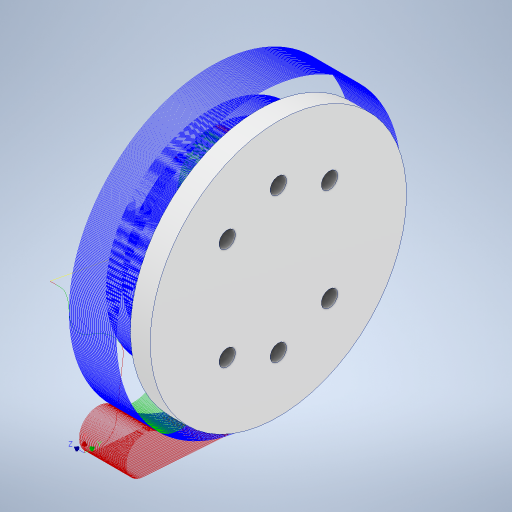
# Autodesk Inventor part: connectpart2
Saved by Autodesk Inventor 2024.3 (Build 283343010, 343A)
## iProperties
Created: 2025-06-26
Part Number: connectpart2
Material: アルミニウム 6061
Document SubType Name: Modeling
Designer: kshau
Density: 2.7 g/cm^3
Appearance: アルミニウム - フラット
Mass: 5.41268 g
Surface Area: 33.3037 cm^2
Volume: 5.41268 cm^3
Author: kshau
Autodesk Inventor part; units mm, degrees
ref_plane "YZ Plane" through (0, 0, 0) normal (1, 0, 0) x (0, 1, 0)
ref_plane "XZ Plane" through (0, 0, 0) normal (0, 1, 0) x (-1, 0, 0)
ref_plane "XY Plane" through (0, 0, 0) normal (0, 0, 1) x (1, 0, 0)
sketch "スケッチ1" plane through (0, 0, 0) normal (1, 0, 0) x (0, 1, 0)
  circle A0 centre (0, 0) radius 19.5
  dimension "d0" = 39
  constraints: 1 centre point, 1 coincident
  measures "d0" diameter of A0
extrude "押し出し1" add sketch "スケッチ1" along normal blind 3
sketch "スケッチ2" plane through (0, 0, 0) normal (-1, 0, 0) x (0, 0, 1)
  circle A0 centre (0, 0) radius 11
  point P0 (0, 11)
  point P1 (-7.7782, 7.7782)
  point P2 (-11, 0)
  point P3 (-7.7782, -7.7782)
  point P4 (0, -11)
  point P5 (7.7782, -7.7782)
  point P6 (11, 0)
  point P7 (7.7782, 7.7782)
  dimension "d3" = 22
  dimension "d6" = 360
  constraints: 1 coincident, 1 vertical alignment, 11 other
hole "穴1" at (0, 7.7782, -7.7782) at (0, 11, 0) at (0, 7.7782, 7.7782) at (0, -7.7782, 7.7782) at (0, -11, 0) at (0, -7.7782, -7.7782) direction (1, 0, 0) diameter 2.5 end through all
sketch "スケッチ3" plane through (3, 0, 0) normal (1, 0, 0) x (0, 0, -1)
  circle A0 centre (-7.7782, 7.7782) radius 1.25 projected
  circle A1 centre (0, 11) radius 1.25 projected
  circle A2 centre (7.7782, 7.7782) radius 1.25 projected
  circle A3 centre (7.7782, -7.7782) radius 1.25 projected
  circle A4 centre (0, -11) radius 1.25 projected
  circle A5 centre (-7.7782, -7.7782) radius 1.25 projected
  point P0 (0, 0)
  constraints: 6 coincident
hole "穴2" [suppressed]
sketch "スケッチ4" plane through (0, 0, 0) normal (-1, 0, 0) x (0, 0, 1)
  circle A0 centre (0, 0) radius 19.5 projected
  circle A1 centre (0, 0) radius 13
  dimension "d22" = 26
  constraints: 1 centre point, 1 coincident
  measures "d22" diameter of A1
extrude "押し出し2" add sketch "スケッチ4" along normal blind 3.8 contours A1
sketch "スケッチ5" plane through (-3.8, 0, 0) normal (-1, 0, 0) x (0, 0, 1)
  point P0 (0, 0)
  point P1 (0, 11)
  point P2 (0, 11)
  point P3 (-7.7782, 7.7782)
  point P4 (-11, 0)
  point P5 (-7.7782, -7.7782)
  point P6 (0, -11)
  point P7 (7.7782, -7.7782)
  point P8 (11, 0)
  point P9 (7.7782, 7.7782)
  dimension "d27" = 360
  constraints: 1 coincident, 9 other
hole "穴3" at (-3.8, 11, 0) at (-3.8, 7.7782, -7.7782) at (-3.8, 7.7782, 7.7782) at (-3.8, -7.7782, 7.7782) at (-3.8, -11, 0) at (-3.8, -7.7782, -7.7782) direction (1, 0, 0) diameter 2.5 end through all
